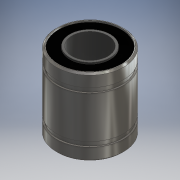
# Autodesk Inventor part: LM8
Saved by Autodesk Inventor 2016 (Build 200138000, 138)
## iProperties
Created: 2016-10-21
Part Number: LM8
Material: Типовые
Document SubType Name: Modeling
Designer: skhalipa
Density: 1 g/cm^3
Appearance: Сталь — полированная
Mass: 3.24799 g
Surface Area: 12.6781 cm^2
Volume: 3.24799 cm^3
Author: skhalipa
Autodesk Inventor part; units mm, degrees
ref_plane "YZ Plane" through (0, 0, 0) normal (1, 0, 0) x (0, 1, 0)
ref_plane "XZ Plane" through (0, 0, 0) normal (0, 1, 0) x (-1, 0, 0)
ref_plane "XY Plane" through (0, 0, 0) normal (0, 0, 1) x (1, 0, 0)
sketch "Эскиз6" plane through (0, 0, 0) normal (0, 0, 1) x (1, 0, 0)
  circle A0 centre (0, 0) radius 7.5
  dimension "d27" = 15
  constraints: 1 centre point, 1 coincident
  measures "d27" diameter of A0
extrude "Выдавливание2" add sketch "Эскиз6" against normal blind 17
sketch "Эскиз8" plane through (0, 0, 0) normal (0, 0, 1) x (1, 0, 0)
  point P0 (0, 0)
  point P1 (0, 0)
  constraints: 1 coincident
hole "Отверстие1" at (0, 0, 0) direction (0, 0, -1) diameter 8 end through all
ref_plane "РабПлоскость1" through (0, 0, -2.75) normal (0, 0, 1) x (1, 0, 0)
ref_plane "РабПлоскость2" through (0, 0, -14.25) normal (0, 0, -1) x (-1, 0, 0)
sketch "Эскиз10" plane through (0, 0, -14.25) normal (0, 0, -1) x (-1, 0, 0)
  circle A0 centre (0, 0) radius 7.15
  circle A1 centre (0, 0) radius 7.5
  dimension "d40" = 14.3
  dimension "d41" = 15
  constraints: 2 centre point, 2 coincident
  measures "d40" diameter of A0
  measures "d41" diameter of A1
sketch "Эскиз11" plane through (0, 0, -2.75) normal (0, 0, 1) x (1, 0, 0)
  circle A0 centre (0, 0) radius 7.15
  circle A1 centre (0, 0) radius 7.5
  dimension "d42" = 14.3
  dimension "d43" = 15
  constraints: 2 centre point, 2 coincident
  measures "d42" diameter of A0
  measures "d43" diameter of A1
extrude "Выдавливание3" cut sketch "Эскиз11" against normal blind 1.1
extrude "Выдавливание4" cut sketch "Эскиз10" against normal blind 1.1
sketch "Эскиз12" plane through (0, 0, -17) normal (0, 0, -1) x (-1, 0, 0)
  circle A0 centre (0, 0) radius 7
  circle A1 centre (0, 0) radius 4.5
  dimension "d48" = 14
  dimension "d49" = 9
  constraints: 2 centre point, 2 coincident
  measures "d48" diameter of A0
  measures "d49" diameter of A1
extrude "Выдавливание5" cut sketch "Эскиз12" against normal blind 0.35
sketch "Эскиз13" plane through (0, 0, 0) normal (0, 0, 1) x (1, 0, 0)
  circle A0 centre (0, 0) radius 4.5
  circle A1 centre (0, 0) radius 7
  dimension "d52" = 9
  dimension "d53" = 14
  constraints: 2 centre point, 2 coincident
  measures "d52" diameter of A0
  measures "d53" diameter of A1
extrude "Выдавливание6" cut sketch "Эскиз13" against normal blind 0.35
chamfer "Фаска1" distance 0.35 angle 45 2 edges at (-7.5, 0, 0) (-7.5, 0, -17)
